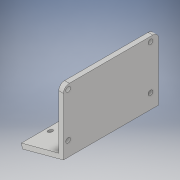
# Autodesk Inventor part: LimeLight120
Saved by Autodesk Inventor 2019 (Build 230136000, 136)
## iProperties
Created: 2019-12-14
Part Number: LimeLight120
Material: Generic
Document SubType Name: Modeling
Designer: james
Density: 1 g/cm^3
Appearance: Default
Author: james
Autodesk Inventor part; units mm, degrees
ref_plane "YZ Plane" through (0, 0, 0) normal (1, 0, 0) x (0, 1, 0)
ref_plane "XZ Plane" through (0, 0, 0) normal (0, 1, 0) x (-1, 0, 0)
ref_plane "XY Plane" through (0, 0, 0) normal (0, 0, 1) x (1, 0, 0)
sketch "Sketch1" plane through (0, 0, 0) normal (1, 0, 0) x (0, 1, 0)
  line L0 (44.4049, 39.363) -> (-19.0951, 39.363)
  line L1 (-19.0951, 39.363) -> (-19.0951, -63.507)
  line L2 (-19.0951, -63.507) -> (44.4049, -63.507)
  line L3 (44.4049, -63.507) -> (44.4049, 39.363)
  point P0 (0, 0)
  dimension "d0" = 102.87
  dimension "d1" = 63.5
  constraints: 8 end point, 2 parallel, 1 horizontal, 1 perpendicular
  measures "d0" distance of L0.end L1.end
  measures "d1" distance of L0.start L0.end
extrude "Extrusion1" add sketch "Sketch1" along normal blind 5.08
sketch "Sketch2" plane through (5.08, 0, 0) normal (1, 0, 0) x (0, 0, -1)
  line L0 (63.507, 44.4049) -> (-39.363, 44.4049) projected
  line L1 (-39.363, 44.4049) -> (-39.363, -19.0951) projected
  point P0 (0, 0)
  point P1 (-34.283, 39.3249)
  point P2 (54.617, 39.3249)
  point P3 (54.617, -8.3001)
  point P4 (-34.283, -8.3001)
  dimension "d4" = 0
  dimension "d5" = 0
  dimension "d6" = 0
  dimension "d7" = 0
  dimension "d8" = 88.9
  dimension "d9" = 5.08
  dimension "d10" = 5.08
  dimension "d11" = 47.625
  measures "d4" horizontal distance of point (-34.283, -8.3) point (-34.283, 39.325)
  measures "d5" horizontal distance of point (54.617, -8.3) point (54.617, 39.325)
  measures "d6" vertical distance of point (-34.283, 39.325) point (54.617, 39.325)
  measures "d7" vertical distance of point (-34.283, -8.3) point (54.617, -8.3)
  measures "d8" distance of point (54.617, 39.325) point (-34.283, 39.325)
  measures "d9" distance from line of L0 point (-34.283, 39.325)
  measures "d10" distance from line of L1 point (-34.283, 39.325)
  measures "d11" distance of point (-34.283, -8.3) point (-34.283, 39.325)
hole "Hole1" at (5.08, 39.3249, 34.283) at (5.08, 39.3249, -54.617) at (5.08, -8.3001, -54.617) at (5.08, -8.3001, 34.283) direction (-1, 0, 0) diameter 5.1054 end through all clearance for "Flat Head Machine Screw (82)" size "#10" standard "Ansi Unified Screw Threads"
fillet "Fillet1" radius 6.35 2 edges at (2.54, 44.4049, 39.363) (2.54, 44.4049, -63.507)
sketch "Sketch7" plane through (0, -19.0951, 39.363) normal (0, 0, 1) x (1, 0, 0)
  line L0 (0, 0) -> (5.08, 0)
  line L1 (5.08, 0) -> (5.08, -5.08)
  line L2 (5.08, -5.08) -> (-39.0821, -16.9132)
  line L3 (-39.0821, -16.9132) -> (-40.3969, -12.0063)
  line L4 (-40.3969, -12.0063) -> (0, -1.182)
  line L5 (0, -1.182) -> (0, 0)
  line L6 (0, 0) -> (5.08, 0) projected
  line L7 (0, 57.15) -> (0, 0) projected
  point P0 (0, 19.0951)
  dimension "d51" = 5.08
  dimension "d52" = 5.08
  dimension "d53" = 105
  dimension "d54" = 5.08
  dimension "d55" = 45.72
  dimension "d56" = 0
  dimension "d57" = 0
  constraints: 12 end point, 3 perpendicular, 1 horizontal, 1 parallel
  measures "d51" distance of L0.start L0.end
  measures "d52" distance of L0.end L1.end
  measures "d53" angle of L2 L1
  measures "d54" distance of L2.end L3.end
  measures "d55" distance of L1.end L2.end
  measures "d56" distance between parallel lines of L0 L6
  measures "d57" distance between parallel lines of L7 L5
extrude "Extrusion4" add sketch "Sketch7" against normal blind 102.87
sketch "Sketch8" plane through (0, -20.2771, 39.363) normal (-0.258819, 0.9659258, 0) x (0.9659258, 0.258819, 0)
  line L0 (0, 0) -> (0, 102.87) projected
  line L1 (-41.822, 0) -> (0, 0) projected
  line L2 (-41.822, 102.87) -> (0, 102.87) projected
  point P0 (5.2481, 39.363)
  point P1 (-10.16, 25.4)
  point P2 (-35.56, 25.4)
  point P3 (-35.56, 76.2)
  point P4 (-10.16, 76.2)
  dimension "d66" = 25.4
  dimension "d67" = 0
  dimension "d68" = 25.4
  dimension "d69" = 0
  dimension "d70" = 50.8
  dimension "d71" = 0
  dimension "d72" = 0
  dimension "d73" = 26.67
  measures "d66" distance from line of point (-10.16, 25.4) L1
  measures "d67" vertical distance of point (-35.56, 25.4) point (-10.16, 25.4)
  measures "d68" distance of point (-10.16, 25.4) point (-35.56, 25.4)
  measures "d69" horizontal distance of point (-35.56, 25.4) point (-35.56, 76.2)
  measures "d70" distance of point (-35.56, 25.4) point (-35.56, 76.2)
  measures "d71" vertical distance of point (-35.56, 76.2) point (-10.16, 76.2)
  measures "d72" horizontal distance of point (-10.16, 76.2) point (-10.16, 25.4)
  measures "d73" distance from line of L2 point (-35.56, 76.2)
hole "Hole3" at (-9.8138, -22.9067, 13.963) at (-34.3483, -29.4807, 13.963) at (-34.3483, -29.4807, -36.837) at (-9.8138, -22.9067, -36.837) direction (0.258819, -0.9659258, 0) diameter 5.1054 end through all clearance for "Flat Head Machine Screw (82)" size "#10" standard "Ansi Unified Screw Threads"
body "Solid1"
